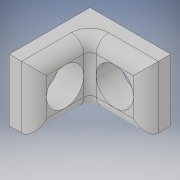
# Autodesk Inventor part: draat tap stukje 1
Saved by Autodesk Inventor 2019 (Build 230136000, 136)
## iProperties
Created: 2021-06-06
Part Number: draat tap stukje 1
Material: Generic
Document SubType Name: Modeling
Designer: Stefan
Density: 1 g/cm^3
Appearance: Default
Author: Stefan
Autodesk Inventor part; units mm, degrees
ref_plane "YZ Plane" through (0, 0, 0) normal (1, 0, 0) x (0, 1, 0)
ref_plane "XZ Plane" through (0, 0, 0) normal (0, 1, 0) x (-1, 0, 0)
ref_plane "XY Plane" through (0, 0, 0) normal (0, 0, 1) x (1, 0, 0)
sketch "Sketch1" plane through (0, 0, 0) normal (0, 0, 1) x (1, 0, 0)
  circle A0 centre (0, 0) radius 1.5
  line L0 (2.5, 2.5) -> (-4, 2.5)
  line L1 (-4, 2.5) -> (-4, -2.5)
  line L2 (-4, -2.5) -> (2.5, -2.5)
  line L3 (2.5, -2.5) -> (2.5, 2.5)
  dimension "d0" = 3
  dimension "d1" = 1
  dimension "d2" = 1
  dimension "d3" = 1
  dimension "d4" = 2.5
  constraints: 8 end point, 2 parallel, 1 centre point, 1 coincident, 1 horizontal, 1 perpendicular
  measures "d0" diameter of A0
  measures "d1" distance edge to line of A0 L0
  measures "d2" distance edge to line of A0 L3
  measures "d3" distance edge to line of A0 L2
  measures "d4" distance edge to line of A0 L1
extrude "Extrusion1" add sketch "Sketch1" along normal blind 2
sketch "Sketch2" plane through (-4, -2.5, 0) normal (-1, 0, 0) x (0, 0, 1)
  line L0 (0, 0) -> (2, 0) projected
  line L1 (0, 0) -> (6.5, 0)
  line L2 (6.5, 0) -> (6.5, 5)
  line L3 (6.5, 5) -> (0, 5)
  line L4 (0, 5) -> (0, 0)
  circle A0 centre (4, 2.5) radius 1.5
  point P0 (0, 2.5)
  dimension "d7" = 3
  dimension "d8" = 2.5
  dimension "d9" = 1
  dimension "d10" = 1
  dimension "d11" = 1
  constraints: 8 end point, 2 parallel, 1 centre point, 1 horizontal, 1 perpendicular
  measures "d7" diameter of A0
  measures "d8" distance edge to line of A0 L4
  measures "d9" distance edge to line of A0 L1
  measures "d10" distance edge to line of A0 L2
  measures "d11" distance edge to line of A0 L3
extrude "Extrusion2" add sketch "Sketch2" against normal blind 2
fillet "Fillet2" radius 0.5 1 edges at (-2, 0, 2)
fillet "Fillet2" radius 1 6 edges at (0.25, 2.5, 2) (-2, 2.5, 4.25) (-2, 0, 6.5) (-2, -2.5, 4.25) (0.25, -2.5, 2) (2.5, 0, 2)
body "Solid1"
